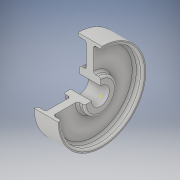
# Autodesk Inventor part: 練習一
Saved by Autodesk Inventor 2017 (Build 210142000, 142)
## iProperties
Part Number: 練習一
Material: 一般
Document SubType Name: Modeling
Designer: user
Density: 1 g/cm^3
Appearance: 預設
Author: user
Autodesk Inventor part; units mm, degrees
ref_plane "YZ Plane" through (0, 0, 0) normal (1, 0, 0) x (0, 1, 0)
ref_plane "XZ Plane" through (0, 0, 0) normal (0, 1, 0) x (-1, 0, 0)
ref_plane "XY Plane" through (0, 0, 0) normal (0, 0, 1) x (1, 0, 0)
sketch "草圖1" plane through (0, 0, 0) normal (0, 0, 1) x (1, 0, 0)
  line L0 (-20, 8.5) -> (0, 8.5)
  line L1 (0, 8.5) -> (0, 15.5)
  line L2 (0, 15.5) -> (-4.5, 15.5)
  line L3 (-6.5, 17.5) -> (-6.5, 37)
  line L4 (-20, 8.5) -> (-20, 15.5)
  line L5 (-4.5, 39) -> (-0.5, 39)
  line L6 (-20, 15.5) -> (-15.5, 15.5)
  line L7 (-13.5, 17.5) -> (-13.5, 37)
  line L8 (-15.5, 39) -> (-19.5, 39)
  line L9 (-21.5, 41) -> (-21.5, 42)
  line L10 (-21.5, 42) -> (1.5, 42)
  line L11 (1.5, 42) -> (1.5, 41)
  arc A0 (-13.5, 37) -> (-15.5, 39) centre (-15.5, 37) ccw
  arc A1 (-4.5, 39) -> (-6.5, 37) centre (-4.5, 37) ccw
  arc A2 (-0.5, 39) -> (1.5, 41) centre (-0.5, 41) ccw
  arc A3 (-21.5, 41) -> (-19.5, 39) centre (-19.5, 41) ccw
  arc A4 (-6.5, 17.5) -> (-4.5, 15.5) centre (-4.5, 17.5) ccw
  arc A5 (-15.5, 15.5) -> (-13.5, 17.5) centre (-15.5, 17.5) ccw
  line L12 (-40.2973, 0) -> (23.5613, 0)
  line L13 (-10, 42) -> (-10, 1.9657)
  point P0 (0, 0)
  point P1 (-6.5, 15.5)
  point P2 (-6.5, 39)
  point P3 (-13.5, 15.5)
  point P4 (-13.5, 39)
  point P5 (-21.5, 39)
  point P6 (1.5, 39)
  dimension "d15" = 0
  dimension "d28" = 23
  dimension "d29" = 7
  dimension "d30" = 20
  dimension "d35" = 84
  dimension "d36" = 78
  dimension "d37" = 17
  dimension "d38" = 31
  dimension "d39" = 0
  dimension "d40" = 31
  dimension "d41" = 78
  dimension "d42" = 8
  dimension "d43" = 2
  dimension "d45" = 20
  constraints: 34 end point, 18 point on line, 12 point on circle, 12 tangent, 7 perpendicular, 6 centre point, 5 equal radius, 4 horizontal, 3 vertical, 1 midpoint
  measures "d15" distance from line of point (0, 0) L1
  measures "d28" distance between parallel lines of L11 L9
  measures "d29" distance between parallel lines of L3 L7
  measures "d30" distance between parallel lines of L1 L4
  measures "d35" diameter of L10 L12
  measures "d36" diameter of L5 L12
  measures "d37" diameter of L0 L12
  measures "d38" diameter of L2 L12
  measures "d39" distance from line of point (0, 0) L12
  measures "d40" diameter of L6 L12
  measures "d41" diameter of L8 L12
  measures "d42" distance between parallel lines of L11 L3
  measures "d43" radius of A5
  measures "d45" diameter of point (0, 0) L13
revolve "迴轉1" add sketch "草圖1" angle 270 about axis through (-40.2973, 0, 0) along (-1, 0, 0)
fillet "圓角3" radius 2 2 edges at (0, -10.9602, -10.9602) (-20, -10.9602, -10.9602)
sketch "草圖11" plane through (0, 8.5, 0) normal (1, 0, 0) x (0, 0, -1)
  point P0 (0, -8.5)
